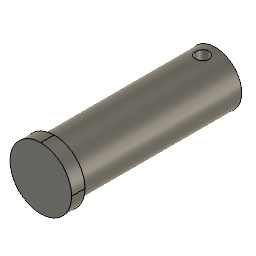
joint_pin (Autodesk Fusion 360 design; units mm, degrees)
part number: 2025-10-30-14-43-40-714
Autodesk Fusion 360 part; units mm, degrees
sketch "Sketch1" plane through (0, 0, 0) normal (0, 1, 0) x (1, 0, 0)
  circle A0 centre (0, -6.35) radius 5.0165
  dimension "d1" = 10.033
  measures "d1" diameter of A0
extrude "Extrude1" add sketch "Sketch1" along normal blind 33.02
hole "Hole1" at (0, 55.245, 11.3665) direction (0, 0, -1) diameter 2.54 depth 19.05 tip angle 118
extrude "Extrude2" cut 1 faces at (-0.3721, 0, 4.7198) along direction (0, 1, 0) blind 2.54
sketch "Sketch3" plane through (0, 2.54, 0) normal (0, -1, 0) x (1, 0, 0)
  circle A0 centre (0, 6.35) radius 5.0165
  line L0 (-2.54, 8.89) -> (2.54, 8.89)
  line L1 (2.54, 8.89) -> (2.54, 3.81)
  line L2 (2.54, 3.81) -> (-2.54, 3.81)
  line L3 (-2.54, 3.81) -> (-2.54, 8.89)
  constraint horizontal L0
  constraint vertical L1
  constraint horizontal L2
  constraint vertical L3
extrude "Extrude3" add sketch "Sketch3" along normal blind 2.54 contours L0 L1 L2 L3
extrude "Extrude4" add 1 faces at (0.8467, 0.8467, 8.89) along direction (0, 0, 1) blind 3.302
extrude "Extrude5" add 1 faces at (2.54, 0.8467, 8.8926) along direction (1, 0, 0) blind 3.302
extrude "Extrude6" add 1 faces at (2.5426, 0.8467, 3.81) along direction (0, 0, -1) blind 3.302
extrude "Extrude7" add 1 faces at (-2.54, 0.8467, 4.908) along direction (-1, 0, 0) blind 3.302
fillet "Fillet1" radius 5.842 4 edges at (-5.842, 1.27, 12.192) (5.842, 1.27, 12.192) (5.842, 1.27, 0.508) (-5.842, 1.27, 0.508)
hole "Hole2" at (0, 30.48, 11.3665) direction (0, 0, -1) diameter 2.54 depth 23.622 tip angle 118
